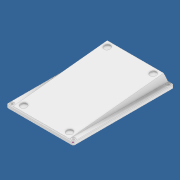
# Autodesk Inventor part: Bottom
Saved by Autodesk Inventor 2020 (Build 240168000, 168)
## iProperties
Created: 2021-08-07
Part Number: Bottom
Material: PC/ABS Plastic
Document SubType Name: Modeling
Designer: RNG3nius
Density: 0.357273 g/cm^3
Appearance: Smooth - White
Author: RNG3nius
Autodesk Inventor part; units mm, degrees
ref_plane "YZ Plane" through (0, 0, 0) normal (1, 0, 0) x (0, 1, 0)
ref_plane "XZ Plane" through (0, 0, 0) normal (0, 1, 0) x (-1, 0, 0)
ref_plane "XY Plane" through (0, 0, 0) normal (0, 0, 1) x (1, 0, 0)
sketch "Sketch1" plane through (0, 0, 0) normal (0, 1, 0) x (-1, 0, 0)
  line L0 (0, 0) -> (63.8, 0)
  line L1 (63.8, 0) -> (63.8, -96)
  line L2 (63.8, -96) -> (0, -96)
  line L3 (0, -96) -> (0, 0)
  dimension "d0" = 63.8
  dimension "d1" = 96
  constraints: 8 end point, 2 parallel, 1 horizontal, 1 perpendicular
  measures "d0" distance of L1.end L2.end
  measures "d1" distance of L0.end L1.end
extrude "Extrusion1" add sketch "Sketch1" along normal blind 3
fillet "Fillet1" radius 1.5 4 edges at (0, 1.5, 0) (0, 1.5, -96) (-63.8, 1.5, -96) (-63.8, 1.5, 0)
sketch "Sketch2" plane through (0, 3, 0) normal (0, 1, 0) x (1, 0, 0)
  circle A0 centre (-2.7, 2.7) radius 1
  circle A1 centre (-61.1, 2.7) radius 1
  circle A2 centre (-61.1, 93.3) radius 1
  circle A3 centre (-2.7, 93.3) radius 1
  line L0 (-1.5, 96) -> (-62.3, 96) projected
  line L1 (0, 1.5) -> (0, 94.5) projected
  line L2 (-63.8, 94.5) -> (-63.8, 1.5) projected
  line L3 (-62.3, 0) -> (-1.5, 0) projected
  point P0 (0, 0)
  dimension "d5" = 2
  dimension "d6" = 2
  dimension "d7" = 2
  dimension "d8" = 2
  dimension "d9" = 2.7
  dimension "d10" = 2.7
  dimension "d11" = 2.7
  dimension "d12" = 2.7
  dimension "d13" = 2.7
  dimension "d14" = 2.7
  dimension "d15" = 2.7
  dimension "d16" = 2.7
  constraints: 4 centre point
  measures "d5" diameter of A0
  measures "d6" diameter of A1
  measures "d7" diameter of A2
  measures "d8" diameter of A3
  measures "d9" distance from line of L0 A3.centre
  measures "d10" distance from line of L1 A3.centre
  measures "d11" distance from line of L2 A2.centre
  measures "d12" distance from line of L0 A2.centre
  measures "d13" distance from line of L2 A1.centre
  measures "d14" distance from line of L3 A1.centre
  measures "d15" distance from line of L3 A0.centre
  measures "d16" distance from line of A0.centre L1
extrude "Extrusion2" cut sketch "Sketch2" against normal blind 10
sketch "Sketch4" plane through (0, 3, 0) normal (0, 1, 0) x (1, 0, 0)
  line L0 (0, 1.5) -> (0, 94.5) projected
  line L1 (-4.5, 1) -> (-58.3, 1)
  line L2 (-58.3, 1) -> (-58.3, 95)
  line L3 (-58.3, 95) -> (-4.5, 95)
  line L4 (-4.5, 95) -> (-4.5, 1)
  line L5 (-62.3, 0) -> (-1.5, 0) projected
  line L6 (-1.5, 96) -> (-62.3, 96) projected
  point P0 (0, 0)
  point P1 (-1.5, 0)
  point P2 (-62.3, 96)
  dimension "d37" = 53.8
  dimension "d38" = 4.5
  dimension "d39" = 95
  dimension "d40" = 95
  constraints: 8 end point, 2 parallel, 1 horizontal, 1 perpendicular, 2 other
  measures "d37" distance of L2.end L3.end
  measures "d38" distance between parallel lines of L0 L4
  measures "d39" distance of the line from the sketch origin of L3
extrude "Extrusion4" add sketch "Sketch4" along normal blind 9.53
sketch "Sketch5" plane through (-58.3, 3, -96) normal (-1, 0, 0) x (0, 0, 1)
  line L0 (1, 9.53) -> (95, 9.53) projected
  line L1 (96, 0) -> (177.6046, 0) construction
  line L2 (96, 0) -> (5.3281, 9.53)
  line L3 (96, 0) -> (187.1713, 0) construction
  line L4 (1, 0) -> (1, 9.53) projected
  line L5 (5.3281, 9.53) -> (1, 0)
  line L6 (5.3281, 9.53) -> (95, 9.53)
  line L7 (95, 0) -> (95, 9.53) projected
  line L8 (96, 0) -> (96, 9.53)
  line L9 (95, 9.53) -> (5.3281, 9.53)
  line L10 (1, 0) -> (1, 9.53) projected
  line L11 (1, 9.53) -> (5.3281, 9.53)
  line L12 (0, -3) -> (0, 0) projected
  line L13 (1, 0) -> (1, 9.53)
  point P0 (96, -3)
  dimension "d44" = 174
  constraints: 18 end point, 2 collinear, 2 horizontal, 1 equal length, 1 parallel, 1 perpendicular, 1 point on line, 1 vertical, 1 other
  measures "d44" angle of L3 L2
extrude "Extrusion5" cut sketch "Sketch5" against normal blind 53.8
sketch "Sketch9" plane through (-58.3, 3, 0) normal (0, 0.9945219, 0.1045285) x (1, 0, 0)
  circle A0 centre (5, 6.0055) radius 3.05
  circle A1 centre (48.8, 6.0055) radius 3.05
  circle A2 centre (48.8, 86.171) radius 3.05
  circle A3 centre (5, 86.171) radius 3.05
  line L0 (53.8, 91.1713) -> (0, 91.1713) projected
  line L1 (0, 1.0055) -> (0, 91.1713) projected
  line L2 (53.8, 91.1713) -> (53.8, 1.0055) projected
  line L3 (53.8, 1.0055) -> (0, 1.0055) projected
  point P0 (58.3, -0.3136)
  point P1 (0, 0)
  point P2 (53.8, 0)
  dimension "d61" = 6.1
  dimension "d62" = 6.1
  dimension "d63" = 6.1
  dimension "d64" = 6.1
  dimension "d65" = 5.0003
  dimension "d66" = 5
  dimension "d67" = 5.0003
  dimension "d68" = 5
  dimension "d69" = 5
  dimension "d70" = 5
  dimension "d71" = 5
  dimension "d72" = 5
  constraints: 4 centre point, 1 other
  measures "d61" diameter of A0
  measures "d62" diameter of A1
  measures "d63" diameter of A2
  measures "d64" diameter of A3
  measures "d65" distance from line of L0 A3.centre
  measures "d66" distance from line of L1 A3.centre
  measures "d67" distance from line of L0 A2.centre
  measures "d68" distance from line of A2.centre L2
  measures "d69" distance from line of L2 A1.centre
  measures "d72" distance from line of L1 A0.centre
extrude "Extrusion8" cut sketch "Sketch9" against normal blind 1 contours A0 | A1 | A2 | A3
sketch "Sketch20" plane through (-58.3, 3, 0) normal (0, 0.9945219, 0.1045285) x (1, 0, 0)
  line L0 (16.9, 89.171) -> (35.9, 89.171)
  line L1 (35.9, 89.171) -> (35.9, 55.171)
  line L2 (35.9, 55.171) -> (16.9, 55.171)
  line L3 (16.9, 55.171) -> (16.9, 89.171)
  line L4 (53.8, 91.1713) -> (0, 91.1713) projected
  line L5 (0, 1.0055) -> (0, 91.1713) projected
  point P0 (58.3, -0.3136)
  point P1 (0, 0)
  dimension "d106" = 19
  dimension "d107" = 34
  dimension "d108" = 2.0003
  dimension "d109" = 16.9
  constraints: 8 end point, 2 parallel, 1 horizontal, 1 perpendicular
  measures "d106" distance of L1.end L2.end
  measures "d107" distance of L0.end L1.end
  measures "d108" distance between parallel lines of L4 L0
  measures "d109" distance between parallel lines of L5 L3
extrude "Extrusion17" cut sketch "Sketch20" against normal blind 18
sketch "Sketch22" plane through (-41.4, 0, -55.7902) normal (1, 0, 0) x (0, 0, -1)
  line L0 (32.8923, 12.3209) -> (34.1873, 0) projected
  line L1 (-0.9214, 8.7669) -> (0, 0) projected
  line L2 (33.2518, 8.9007) -> (-0.562, 5.3467)
  line L3 (-0.562, 5.3467) -> (-0.9214, 8.7669)
  line L4 (-0.9214, 8.7669) -> (32.8923, 12.3209) projected
  line L5 (-0.9214, 8.7669) -> (32.8923, 12.3209)
  line L6 (32.8923, 12.3209) -> (33.2518, 8.9007)
  point P0 (-55.7902, 0)
  dimension "d116" = 3.4391
  constraints: 8 end point, 2 perpendicular, 2 point on line, 1 collinear
  measures "d116" distance between parallel lines of L4 L2
extrude "Extrusion19" add sketch "Sketch22" along normal blind 19
sketch "Sketch24" plane through (-41.4, 5.3467, -55.2282) normal (0, -0.9945219, -0.1045285) x (1, 0, 0)
  line L0 (20, -35) -> (0, -35)
  line L1 (0, 0) -> (19, 0)
  line L2 (0, -34) -> (0, 0) projected
  line L3 (0, 0) -> (19, 0)
  line L4 (19, 0) -> (19, -34)
  line L5 (19, -34) -> (0, -34)
  line L6 (0, -34) -> (0, 0)
  point P0 (41.4, 55.4846)
  point P1 (0, -34)
  constraints: 12 end point, 2 horizontal, 2 parallel, 1 perpendicular
extrude "Extrusion21" cut sketch "Sketch24" against normal blind 1 from surface at 0
sketch "Sketch29" plane through (0, 3, 0) normal (0, 1, 0) x (1, 0, 0)
  circle A0 centre (-2.7, 2.7) radius 1 projected
  circle A1 centre (-2.7, 2.7) radius 2
  circle A2 centre (-2.7, 93.3) radius 1 projected
  circle A3 centre (-2.7, 93.3) radius 2
  circle A4 centre (-61.1, 2.7) radius 1 projected
  circle A5 centre (-61.1, 2.7) radius 2
  circle A6 centre (-61.1, 93.3) radius 1 projected
  circle A7 centre (-61.1, 93.3) radius 2
  point P0 (0, 0)
  dimension "d137" = 4
  dimension "d138" = 4
  dimension "d139" = 4
  dimension "d141" = 4
  constraints: 4 centre point, 4 coincident
  measures "d137" diameter of A1
  measures "d138" diameter of A3
  measures "d139" diameter of A5
  measures "d141" diameter of A7
extrude "Extrusion24" cut sketch "Sketch29" against normal blind 0.3 contours A1 | A2 | A3 | A4 | A5 | A6 | A7
ref_plane "Work Plane4" through (-41.4, 8.9007, -89.042) normal (0, -0.1045285, 0.9945219) x (1, 0, 0)
sketch "Sketch31" plane through (-41.4, 8.9007, -89.042) normal (0, -0.1045285, 0.9945219) x (1, 0, 0)
  line L0 (20, 0) -> (0, 0) projected
  line L1 (5, 0) -> (15, 0)
  line L2 (15, 0) -> (15, -4)
  line L3 (15, -4) -> (5, -4)
  line L4 (5, -4) -> (5, 0)
  line L5 (0, -9.3721) -> (0, 0) projected
  point P0 (41.4, 0.4555)
  dimension "d144" = 10
  dimension "d145" = 4
  dimension "d146" = 5
  constraints: 8 end point, 2 parallel, 1 horizontal, 1 perpendicular, 1 point on line
  measures "d144" distance of L2.end L3.end
  measures "d145" distance of L1.end L2.end
  measures "d146" distance between parallel lines of L5 L4
extrude "Extrusion25" cut sketch "Sketch31" against normal blind 20
ref_plane "Work Plane5" through (-40.9, 11.045, -99.8772) normal (0, -0.1045285, 0.9945219) x (1, 0, 0)
sketch "Sketch33" plane through (-40.9, 11.045, -99.8772) normal (0, -0.1045285, 0.9945219) x (1, 0, 0)
  line L0 (1.5, 1.2498) -> (17.5, 1.2498)
  line L1 (17.5, 1.2498) -> (17.5, -7.2502)
  line L2 (17.5, -7.2502) -> (1.5, -7.2502)
  line L3 (1.5, -7.2502) -> (1.5, 1.2498)
  line L4 (36.4, -7.5956) -> (36.4, 2.4391) projected
  line L5 (39.4, -10.5792) -> (-21.4, -10.5792) projected
  point P0 (40.9, -0.5445)
  dimension "d157" = 16
  dimension "d158" = 8.5
  dimension "d159" = 18.9
  dimension "d160" = 3.329
  constraints: 8 end point, 2 parallel, 1 horizontal, 1 perpendicular
  measures "d157" distance of L1.end L2.end
  measures "d158" distance of L0.end L1.end
  measures "d159" distance between parallel lines of L4 L1
  measures "d160" distance between parallel lines of L5 L2
extrude "Extrusion27" cut sketch "Sketch33" along normal blind 10
fillet "Fillet5" radius 2 4 edges at (-26.4, 8.9528, -89.5383) (-26.4, 4.9747, -89.9564) (-36.4, 8.9528, -89.5383) (-36.4, 4.9747, -89.9564)
fillet "Fillet7" radius 4.24 4 edges at (-39.4, 3.0101, -92.7914) (-39.4, 11.3155, -90.4948) (-23.4, 3.0101, -92.7914) (-23.4, 11.3155, -90.4948)
sketch "Sketch34" plane through (-41.4, 6.3412, -55.1237) normal (0, -0.9945219, -0.1045285) x (1, 0, 0)
  line L0 (0, 0) -> (19, 0) projected
  line L1 (19, -34) -> (0, -34) projected
  line L2 (19, 0) -> (16, 0)
  line L3 (16, 0) -> (16, -34)
  line L4 (16, -34) -> (19, -34)
  line L5 (19, -34) -> (19, 0)
  line L6 (0, -34) -> (0, 0) projected
  line L7 (0, 0) -> (3, 0)
  line L8 (3, 0) -> (3, -34)
  line L9 (3, -34) -> (0, -34)
  line L10 (0, -34) -> (0, 0)
  point P0 (41.4, 55.4846)
  point P1 (19, -34)
  point P2 (16, 0)
  point P3 (3, -34)
  point P4 (3, 0)
  dimension "d167" = 3
  dimension "d168" = 3
  constraints: 16 end point, 4 parallel, 2 horizontal, 2 perpendicular, 2 point on line
  measures "d167" distance of L4.end L3.end
  measures "d168" distance of L8.end L9.end
extrude "Extrusion28" cut sketch "Sketch34" against normal blind 1 contours L0 L8 L1 L6 | L0 L5 L1 L3
sketch "Sketch35" plane through (-58.3, 3, 0) normal (0, 0.9945219, 0.1045285) x (1, 0, 0)
  point P0 (58.3, -0.3136)
chamfer "Chamfer2" distance 0.5 angle 45 8 edges at (-63.8, 3, -48) (-63.3607, 3, -0.4393) (-31.9, 3, 0) (-0.4393, 3, -0.4393) (0, 3, -48) (-0.4393, 3, -95.5607) (-31.9, 3, -96) (-63.3607, 3, -95.5607)
body "Solid1"
